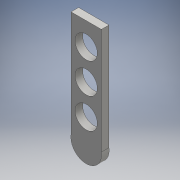
# Autodesk Inventor part: trainingwheels
Saved by Autodesk Inventor 2016 (Build 200138000, 138)
## iProperties
Created: 2016-03-20
Part Number: trainingwheels
Material: Generic
Document SubType Name: Modeling
Designer: mkepler
Density: 1 g/cm^3
Appearance: Default
Author: mkepler
Autodesk Inventor part; units mm, degrees
ref_plane "YZ Plane" through (0, 0, 0) normal (1, 0, 0) x (0, 1, 0)
ref_plane "XZ Plane" through (0, 0, 0) normal (0, 1, 0) x (-1, 0, 0)
ref_plane "XY Plane" through (0, 0, 0) normal (0, 0, 1) x (1, 0, 0)
sketch "Sketch1" plane through (0, 0, 0) normal (0, 1, 0) x (-1, 0, 0)
  line L0 (0, 0) -> (6, 0)
  line L1 (6, 0) -> (6, -21)
  line L2 (0, -21) -> (0, 0)
  circle A0 centre (3, -4.5) radius 2.2
  circle A1 centre (3, -10.5) radius 2.2
  circle A2 centre (3, -16.5) radius 2.2
  arc A3 (0, -21) -> (6, -21) centre (3, -21.4682) ccw
  dimension "d0" = 6
  dimension "d1" = 21
  dimension "d2" = 4.4
  dimension "d3" = 3
  dimension "d4" = 4.5
  dimension "d5" = 4.4
  dimension "d6" = 6
  dimension "d7" = 4.4
  dimension "d8" = 6
  constraints: 6 end point, 4 centre point, 2 point on circle, 1 horizontal, 1 parallel, 1 perpendicular
  measures "d0" distance of L1.end L2.start
  measures "d1" distance of L0.end L1.end
  measures "d2" diameter of A0
  measures "d3" distance from line of L1 A0.centre
  measures "d4" distance from line of L0 A0.centre
  measures "d5" diameter of A1
  measures "d6" distance of A0.centre A1.centre
  measures "d7" diameter of A2
  measures "d8" distance of A2.centre A1.centre
extrude "Extrusion1" add sketch "Sketch1" along normal blind 1.5
body "Solid1"
